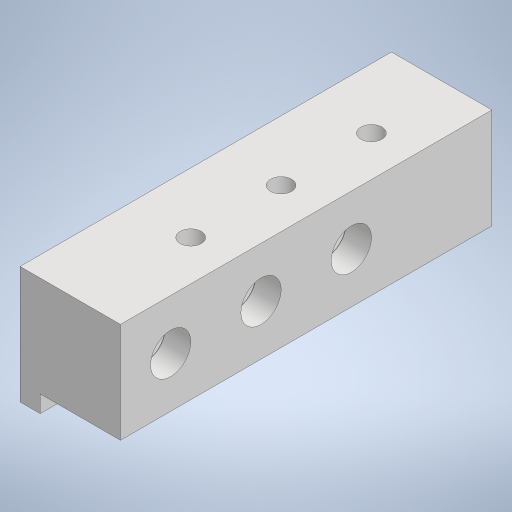
# Autodesk Inventor part: probe_mount
Saved by Autodesk Inventor 2024.1 (Build 281209000, 209)
## iProperties
Created: 2023-10-07
Part Number: probe_mount
Material: Generic
Document SubType Name: Modeling
Designer: l1534
Density: 1 g/cm^3
Appearance: Default
Author: l1534
Autodesk Inventor part; units mm, degrees
ref_plane "YZ Plane" through (0, 0, 0) normal (1, 0, 0) x (0, 1, 0)
ref_plane "XZ Plane" through (0, 0, 0) normal (0, 1, 0) x (-1, 0, 0)
ref_plane "XY Plane" through (0, 0, 0) normal (0, 0, 1) x (1, 0, 0)
sketch "Sketch1" plane through (0, 0, 0) normal (1, 0, 0) x (0, 1, 0)
  line L0 (12.0648, 10.4185) -> (22.0648, 10.4185)
  line L1 (22.0648, 10.4185) -> (22.0648, -17.5815)
  line L2 (22.0648, -17.5815) -> (12.0648, -17.5815)
  line L3 (12.0648, -17.5815) -> (12.0648, 10.4185)
  point P0 (0, 0)
  dimension "d0" = 28
  dimension "d1" = 10
  constraints: 8 end point, 2 parallel, 1 horizontal, 1 perpendicular
  measures "d0" distance of L0.end L1.end
  measures "d1" distance of L0.start L0.end
extrude "Extrusion1" add sketch "Sketch1" along normal blind 10
sketch "Sketch2" plane through (0, 12.0648, -17.5815) normal (0, -1, 0) x (1, 0, 0)
  line L0 (0, 28) -> (10, 28) projected
  line L1 (0, 0) -> (10, 0) projected
  line L2 (0, 28) -> (2, 28)
  line L3 (2, 28) -> (2, 0)
  line L4 (2, 0) -> (0, 0)
  line L5 (0, 0) -> (0, 28)
  point P0 (0, 17.5815)
  dimension "d4" = 2
  constraints: 8 end point, 2 parallel, 1 horizontal, 1 perpendicular, 1 point on line
  measures "d4" distance between parallel lines of L5 L3
extrude "Extrusion2" add sketch "Sketch2" along normal blind 1.7
sketch "Sketch3" plane through (10, 12.0648, -17.5815) normal (0, -1, 0) x (1, 0, 0)
  circle A0 centre (-4, 8) radius 1.05
  circle A1 centre (-4, 17) radius 1.05
  line L0 (-8, 0) -> (0, 0) projected
  line L1 (-8, 0) -> (-8, 28) projected
  point P0 (-10, 17.5815)
  dimension "d7" = 2.1
  dimension "d8" = 2.1
  dimension "d9" = 8
  dimension "d10" = 9
  dimension "d11" = 4
  dimension "d12" = 4
  constraints: 2 centre point
  measures "d7" diameter of A1
  measures "d8" diameter of A0
  measures "d9" distance from line of L0 A0.centre
  measures "d10" distance of A1.centre A0.centre
  measures "d11" distance from line of L1 A0.centre
  measures "d12" distance from line of L1 A1.centre
extrude "Extrusion3" cut sketch "Sketch3" against normal through all
sketch "Sketch4" plane through (10, 0, 0) normal (1, 0, 0) x (0, 0, -1)
  circle A0 centre (-5.4185, 17.0648) radius 1.05
  circle A1 centre (3.5815, 17.0648) radius 1.05
  circle A2 centre (12.5815, 17.0648) radius 1.05
  line L0 (17.5815, 22.0648) -> (-10.4185, 22.0648) projected
  line L1 (17.5815, 12.0648) -> (17.5815, 22.0648) projected
  point P0 (0, 0)
  dimension "d15" = 2.1
  dimension "d16" = 2.1
  dimension "d17" = 2.1
  dimension "d18" = 5
  dimension "d19" = 5
  dimension "d20" = 5
  dimension "d21" = 5
  dimension "d22" = 9
  dimension "d23" = 9
  constraints: 3 centre point
  measures "d15" diameter of A0
  measures "d16" diameter of A1
  measures "d17" diameter of A2
  measures "d18" distance from line of L0 A0.centre
  measures "d19" distance from line of L0 A1.centre
  measures "d20" distance from line of L0 A2.centre
  measures "d21" distance from line of L1 A2.centre
  measures "d22" distance of A2.centre A1.centre
  measures "d23" distance of A1.centre A0.centre
extrude "Extrusion4" cut sketch "Sketch4" against normal through all
sketch "Sketch5" plane through (10, 0, 0) normal (1, 0, 0) x (0, 0, -1)
  circle A0 centre (-5.4185, 17.0648) radius 1.05 projected
  circle A1 centre (-5.4185, 17.0648) radius 2
  circle A2 centre (3.5815, 17.0648) radius 1.05 projected
  circle A3 centre (3.5815, 17.0648) radius 2
  circle A4 centre (12.5815, 17.0648) radius 1.05 projected
  circle A5 centre (12.5815, 17.0648) radius 2
  point P0 (0, 0)
  dimension "d26" = 4
  dimension "d27" = 4
  dimension "d28" = 4
  constraints: 3 centre point, 3 coincident
  measures "d26" diameter of A5
  measures "d27" diameter of A3
  measures "d28" diameter of A1
extrude "Extrusion5" cut sketch "Sketch5" against normal blind 2.5
chamfer "Chamfer1" distance 0.9 angle 45 3 edges at (7.5, 17.0648, 6.4685) (7.5, 17.0648, -2.5315) (7.5, 17.0648, -11.5315)
sketch "Sketch6" plane through (10, 22.0648, -17.5815) normal (0, 0, -1) x (-1, 0, 0)
  line L0 (0, 0) -> (0, -10) projected
  line L1 (0, -10) -> (0, 0)
  line L2 (0, 0) -> (10, 0)
  line L3 (8, -11.7) -> (10, -11.7) projected
  line L4 (10, 0) -> (10, -11.7)
  line L5 (8, -11.7) -> (8, -10)
  line L6 (8, -10) -> (0, -10)
  point P0 (10, -22.0648)
  constraints: 10 end point, 2 perpendicular, 2 vertical, 1 horizontal
extrude "Extrusion6" add sketch "Sketch6" along normal blind 9
sketch "Sketch7" plane through (2, 12.0648, 10.4185) normal (0, -1, 0) x (1, 0, 0)
  circle A0 centre (4, -29) radius 1.05
  line L0 (0, 0) -> (0, -37) projected
  line L1 (8, -37) -> (0, -37) projected
  point P0 (-2, -10.4185)
  dimension "d39" = 2.1
  dimension "d40" = 4
  dimension "d41" = 8
  constraints: 1 centre point
  measures "d39" diameter of A0
  measures "d40" distance from line of L0 A0.centre
  measures "d41" distance from line of L1 A0.centre
extrude "Extrusion7" cut sketch "Sketch7" against normal through all
body "Solid1"
